Autodesk Fusion 360 part; units mm, degrees
note: some values were not read from the file. Chosen so that the rebuilt part matches the saved one: which bodies a step acts on.
(part 2 of 2)
sketch "Sketch6" plane through (0, 3, 0) normal (0, 1, 0) x (-1, 0, 0)
  line L0 (-6.1781, 100.7305) -> (-1.9988, 100.5953)
  line L1 (-1.9988, 100.5953) -> (-0.8032, 103.5868)
  line L2 (-0.8032, 103.5868) -> (0.6012, 103.5414)
  line L3 (0.6012, 103.5414) -> (-3.5606, 93.6708)
  line L4 (-3.5606, 93.6708) -> (-4.9855, 93.717)
  line L5 (-4.9855, 93.717) -> (-8.7527, 103.8441)
  line L6 (-8.7527, 103.8441) -> (-7.246, 103.7953)
  line L7 (-7.246, 103.7953) -> (-6.1781, 100.7305)
  spline S0 degree 2 poles (18.1316, 102.5774) (18.5781, 102.8912) (19.2412, 103.038) knots 0 0 0 1 1 1
  spline S1 degree 2 poles (19.2412, 103.038) (19.9043, 103.1848) (20.8588, 103.1554) knots 0 0 0 1 1 1
  line L8 (20.8588, 103.1554) -> (24.6701, 103.0379)
  line L9 (24.6701, 103.0379) -> (24.3621, 93.0427)
  line L10 (24.3621, 93.0427) -> (20.6122, 93.1582)
  spline S2 degree 2 poles (20.6122, 93.1582) (19.4667, 93.1935) (18.784, 93.5182) knots 0 0 0 1 1 1
  spline S3 degree 2 poles (18.784, 93.5182) (18.1014, 93.843) (17.7288, 94.4857) knots 0 0 0 1 1 1
  spline S4 degree 2 poles (17.7288, 94.4857) (17.3562, 95.1285) (17.3774, 95.8171) knots 0 0 0 1 1 1
  spline S5 degree 2 poles (17.3774, 95.8171) (17.3971, 96.458) (17.7623, 97.0132) knots 0 0 0 1 1 1
  spline S6 degree 2 poles (17.7623, 97.0132) (18.1274, 97.5683) (18.8404, 97.8944) knots 0 0 0 1 1 1
  spline S7 degree 2 poles (18.8404, 97.8944) (17.9418, 98.1883) (17.4741, 98.8442) knots 0 0 0 1 1 1
  spline S8 degree 2 poles (17.4741, 98.8442) (17.0063, 99.5001) (17.0332, 100.3728) knots 0 0 0 1 1 1
  spline S9 degree 2 poles (17.0332, 100.3728) (17.0548, 101.0751) (17.37, 101.6693) knots 0 0 0 1 1 1
  spline S10 degree 2 poles (17.37, 101.6693) (17.6852, 102.2636) (18.1316, 102.5774) knots 0 0 0 1 1 1
  line L11 (9.2769, 96.8199) -> (3.1378, 96.8199)
  line L12 (3.1378, 96.8199) -> (3.1378, 98)
  line L13 (3.1378, 98) -> (10.6003, 98)
  line L14 (10.6003, 98) -> (10.6003, 88)
  line L15 (10.6003, 88) -> (3.3697, 88)
  line L16 (3.3697, 88) -> (3.3697, 89.1801)
  line L17 (3.3697, 89.1801) -> (9.2769, 89.1801)
  line L18 (9.2769, 89.1801) -> (9.2769, 92.2428)
  line L19 (9.2769, 92.2428) -> (3.7449, 92.2428)
  line L20 (3.7449, 92.2428) -> (3.7449, 93.4161)
  line L21 (3.7449, 93.4161) -> (9.2769, 93.4161)
  line L22 (9.2769, 93.4161) -> (9.2769, 96.8199)
  circle A0 centre (0, 10) radius 1.5
  circle A1 centre (18.755, -13.3979) radius 1.5
  circle A2 centre (-50, 20) radius 1.5
  circle A3 centre (50, 10) radius 1.5
  circle A4 centre (19.4752, -45.0876) radius 1.5
  circle A5 centre (30, -66.3341) radius 1.5
  circle A6 centre (50, 80) radius 1.5
  circle A7 centre (-20, 20) radius 1.5
  circle A8 centre (-20.1369, -46.1679) radius 1.5
  circle A9 centre (-29.8599, -66.6942) radius 1.5
  circle A10 centre (0, 80) radius 1.5
  circle A11 centre (-20.8571, -13.7581) radius 1.5
  arc A12 (60, 0) -> (30, -30) centre (60, -30) ccw
  line L23 (60, 0) -> (60, 60)
  line L24 (60, 60) -> (70, 70)
  line L25 (70, 70) -> (70, 110)
  line L26 (70, 110) -> (-70, 110)
  line L27 (-70, 110) -> (-70, 70)
  line L28 (-70, 70) -> (-60, 60)
  line L29 (-60, 60) -> (-60, 0)
  arc A13 (-30, -30) -> (-60, 0) centre (-60, -30) ccw
  line L30 (-30, -30) -> (-30, -60)
  line L31 (-30, -60) -> (-60, -40)
  line L32 (-60, -40) -> (-60, -80)
  line L33 (-60, -80) -> (-30, -80)
  line L34 (-30, -80) -> (0, -100)
  line L35 (0, -100) -> (30, -80)
  line L36 (30, -80) -> (60, -80)
  line L37 (60, -80) -> (60, -40)
  line L38 (60, -40) -> (30, -60)
  line L39 (30, -60) -> (30, -30)
  line L40 (-15.3458, 97.2305) -> (-13.811, 97.2305)
  line L41 (-13.811, 97.2305) -> (-13.811, 101.6712)
  line L42 (-13.811, 101.6712) -> (-12.4876, 101.6712)
  line L43 (-12.4876, 101.6712) -> (-12.4876, 91.6712)
  line L44 (-12.4876, 91.6712) -> (-16.9215, 91.6712)
  spline S11 degree 2 poles (-16.9215, 91.6712) (-18.2585, 91.6712) (-18.9542, 91.9406) knots 0 0 0 1 1 1
  spline S12 degree 2 poles (-18.9542, 91.9406) (-19.65, 92.2101) (-20.0661, 92.8922) knots 0 0 0 1 1 1
  spline S13 degree 2 poles (-20.0661, 92.8922) (-20.4822, 93.5743) (-20.4822, 94.3997) knots 0 0 0 1 1 1
  spline S14 degree 2 poles (-20.4822, 94.3997) (-20.4822, 95.4638) (-19.7932, 96.1937) knots 0 0 0 1 1 1
  spline S15 degree 2 poles (-19.7932, 96.1937) (-19.1043, 96.9236) (-17.665, 97.1214) knots 0 0 0 1 1 1
  spline S16 degree 2 poles (-17.665, 97.1214) (-18.1902, 97.3738) (-18.4631, 97.6193) knots 0 0 0 1 1 1
  spline S17 degree 2 poles (-18.4631, 97.6193) (-19.0429, 98.1514) (-19.5613, 98.9495) knots 0 0 0 1 1 1
  line L45 (-19.5613, 98.9495) -> (-21.3007, 101.6712)
  line L46 (-21.3007, 101.6712) -> (-19.6364, 101.6712)
  line L47 (-19.6364, 101.6712) -> (-18.313, 99.5907)
  spline S18 degree 2 poles (-18.313, 99.5907) (-17.7332, 98.6903) (-17.358, 98.2128) knots 0 0 0 1 1 1
  spline S19 degree 2 poles (-17.358, 98.2128) (-16.9829, 97.7353) (-16.6861, 97.5443) knots 0 0 0 1 1 1
  spline S20 degree 2 poles (-16.6861, 97.5443) (-16.3894, 97.3533) (-16.0825, 97.2783) knots 0 0 0 1 1 1
  spline S21 degree 2 poles (-16.0825, 97.2783) (-15.8574, 97.2305) (-15.3458, 97.2305) knots 0 0 0 1 1 1
  line L48 (-24.0007, 95.7872) -> (-25.249, 95.6779)
  spline S22 degree 2 poles (-25.249, 95.6779) (-25.3378, 96.4282) (-25.6618, 96.9091) knots 0 0 0 1 1 1
  spline S23 degree 2 poles (-25.6618, 96.9091) (-25.9859, 97.39) (-26.6681, 97.6866) knots 0 0 0 1 1 1
  spline S24 degree 2 poles (-26.6681, 97.6866) (-27.3502, 97.9833) (-28.2029, 97.9832) knots 0 0 0 1 1 1
  spline S25 degree 2 poles (-28.2029, 97.9832) (-28.96, 97.9831) (-29.5398, 97.7579) knots 0 0 0 1 1 1
  spline S26 degree 2 poles (-29.5398, 97.7579) (-30.1196, 97.5328) (-30.4027, 97.1405) knots 0 0 0 1 1 1
  spline S27 degree 2 poles (-30.4027, 97.1405) (-30.6857, 96.7483) (-30.6856, 96.2844) knots 0 0 0 1 1 1
  spline S28 degree 2 poles (-30.6856, 96.2844) (-30.6856, 95.8137) (-30.4127, 95.4625) knots 0 0 0 1 1 1
  spline S29 degree 2 poles (-30.4127, 95.4625) (-30.1398, 95.1112) (-29.5122, 94.8725) knots 0 0 0 1 1 1
  spline S30 degree 2 poles (-29.5122, 94.8725) (-29.1098, 94.7157) (-27.7318, 94.385) knots 0 0 0 1 1 1
  spline S31 degree 2 poles (-27.7318, 94.385) (-26.3539, 94.0543) (-25.8013, 93.7611) knots 0 0 0 1 1 1
  spline S32 degree 2 poles (-25.8013, 93.7611) (-25.0851, 93.386) (-24.7337, 92.8301) knots 0 0 0 1 1 1
  spline S33 degree 2 poles (-24.7337, 92.8301) (-24.3823, 92.2742) (-24.3823, 91.5852) knots 0 0 0 1 1 1
  spline S34 degree 2 poles (-24.3823, 91.5852) (-24.3822, 90.8281) (-24.8119, 90.1698) knots 0 0 0 1 1 1
  spline S35 degree 2 poles (-24.8119, 90.1698) (-25.2415, 89.5115) (-26.0669, 89.1703) knots 0 0 0 1 1 1
  spline S36 degree 2 poles (-26.0669, 89.1703) (-26.8922, 88.8292) (-27.9018, 88.829) knots 0 0 0 1 1 1
  spline S37 degree 2 poles (-27.9018, 88.829) (-29.0136, 88.8289) (-29.8629, 89.187) knots 0 0 0 1 1 1
  spline S38 degree 2 poles (-29.8629, 89.187) (-30.7122, 89.545) (-31.1693, 90.2407) knots 0 0 0 1 1 1
  spline S39 degree 2 poles (-31.1693, 90.2407) (-31.6264, 90.9364) (-31.6606, 91.8164) knots 0 0 0 1 1 1
  line L49 (-31.6606, 91.8164) -> (-30.3919, 91.912)
  spline S40 degree 2 poles (-30.3919, 91.912) (-30.2894, 90.9639) (-29.6993, 90.4796) knots 0 0 0 1 1 1
  spline S41 degree 2 poles (-29.6993, 90.4796) (-29.1092, 89.9954) (-27.9565, 89.9955) knots 0 0 0 1 1 1
  spline S42 degree 2 poles (-27.9565, 89.9955) (-26.7559, 89.9956) (-26.2068, 90.4356) knots 0 0 0 1 1 1
  spline S43 degree 2 poles (-26.2068, 90.4356) (-25.6578, 90.8757) (-25.6578, 91.4964) knots 0 0 0 1 1 1
  spline S44 degree 2 poles (-25.6578, 91.4964) (-25.6579, 92.0353) (-26.0468, 92.3831) knots 0 0 0 1 1 1
  spline S45 degree 2 poles (-26.0468, 92.3831) (-26.4288, 92.731) (-28.0421, 93.0957) knots 0 0 0 1 1 1
  spline S46 degree 2 poles (-28.0421, 93.0957) (-29.6553, 93.4605) (-30.2556, 93.7333) knots 0 0 0 1 1 1
  spline S47 degree 2 poles (-30.2556, 93.7333) (-31.1288, 94.1357) (-31.545, 94.7529) knots 0 0 0 1 1 1
  spline S48 degree 2 poles (-31.545, 94.7529) (-31.9611, 95.3702) (-31.9612, 96.1751) knots 0 0 0 1 1 1
  spline S49 degree 2 poles (-31.9612, 96.1751) (-31.9613, 96.9732) (-31.5043, 97.6793) knots 0 0 0 1 1 1
  spline S50 degree 2 poles (-31.5043, 97.6793) (-31.0474, 98.3853) (-30.1914, 98.7776) knots 0 0 0 1 1 1
  spline S51 degree 2 poles (-30.1914, 98.7776) (-29.3353, 99.17) (-28.2644, 99.1701) knots 0 0 0 1 1 1
  spline S52 degree 2 poles (-28.2644, 99.1701) (-26.907, 99.1702) (-25.9895, 98.7747) knots 0 0 0 1 1 1
  spline S53 degree 2 poles (-25.9895, 98.7747) (-25.072, 98.3791) (-24.55, 97.5845) knots 0 0 0 1 1 1
  spline S54 degree 2 poles (-24.55, 97.5845) (-24.0281, 96.7899) (-24.0007, 95.7872) knots 0 0 0 1 1 1
extrude "Extrude6" cut sketch "Sketch6" against normal blind 3 contours L48 S22 S23 S24 S25 S26 S27 S28 S29 S30 S31 S32 S33 S34 S35 S36 S37 S38 S39 L49 S40 S41 S42 S43 S44 S45 S46 S47 S48 S49 S50 S51 S52 S53 S54 bodies 10
sketch "Sketch7" plane through (0, 3, 0) normal (0, 1, 0) x (-1, 0, 0)
  spline S0 degree 2 poles (-28.2644, 99.1701) (-26.907, 99.1702) (-25.9895, 98.7747) knots 0 0 0 1 1 1
  spline S1 degree 2 poles (-25.9895, 98.7747) (-25.072, 98.3791) (-24.55, 97.5845) knots 0 0 0 1 1 1
  spline S2 degree 2 poles (-24.55, 97.5845) (-24.0281, 96.7899) (-24.0007, 95.7872) knots 0 0 0 1 1 1
  line L0 (-24.0007, 95.7872) -> (-25.249, 95.6779)
  spline S3 degree 2 poles (-25.249, 95.6779) (-25.3378, 96.4282) (-25.6618, 96.9091) knots 0 0 0 1 1 1
  spline S4 degree 2 poles (-25.6618, 96.9091) (-25.9859, 97.39) (-26.6681, 97.6866) knots 0 0 0 1 1 1
  spline S5 degree 2 poles (-26.6681, 97.6866) (-27.3502, 97.9833) (-28.2029, 97.9832) knots 0 0 0 1 1 1
  spline S6 degree 2 poles (-28.2029, 97.9832) (-28.96, 97.9831) (-29.5398, 97.7579) knots 0 0 0 1 1 1
  spline S7 degree 2 poles (-29.5398, 97.7579) (-30.1196, 97.5328) (-30.4027, 97.1405) knots 0 0 0 1 1 1
  spline S8 degree 2 poles (-30.4027, 97.1405) (-30.6857, 96.7483) (-30.6856, 96.2844) knots 0 0 0 1 1 1
  spline S9 degree 2 poles (-30.6856, 96.2844) (-30.6856, 95.8137) (-30.4127, 95.4625) knots 0 0 0 1 1 1
  spline S10 degree 2 poles (-30.4127, 95.4625) (-30.1398, 95.1112) (-29.5122, 94.8725) knots 0 0 0 1 1 1
  spline S11 degree 2 poles (-29.5122, 94.8725) (-29.1098, 94.7157) (-27.7318, 94.385) knots 0 0 0 1 1 1
  spline S12 degree 2 poles (-27.7318, 94.385) (-26.3539, 94.0543) (-25.8013, 93.7611) knots 0 0 0 1 1 1
  spline S13 degree 2 poles (-25.8013, 93.7611) (-25.0851, 93.386) (-24.7337, 92.8301) knots 0 0 0 1 1 1
  spline S14 degree 2 poles (-24.7337, 92.8301) (-24.3823, 92.2742) (-24.3823, 91.5852) knots 0 0 0 1 1 1
  spline S15 degree 2 poles (-24.3823, 91.5852) (-24.3822, 90.8281) (-24.8119, 90.1698) knots 0 0 0 1 1 1
  spline S16 degree 2 poles (-24.8119, 90.1698) (-25.2415, 89.5115) (-26.0669, 89.1703) knots 0 0 0 1 1 1
  spline S17 degree 2 poles (-26.0669, 89.1703) (-26.8922, 88.8292) (-27.9018, 88.829) knots 0 0 0 1 1 1
  spline S18 degree 2 poles (-27.9018, 88.829) (-29.0136, 88.8289) (-29.8629, 89.187) knots 0 0 0 1 1 1
  spline S19 degree 2 poles (-29.8629, 89.187) (-30.7122, 89.545) (-31.1693, 90.2407) knots 0 0 0 1 1 1
  spline S20 degree 2 poles (-31.1693, 90.2407) (-31.6264, 90.9364) (-31.6606, 91.8164) knots 0 0 0 1 1 1
  line L1 (-31.6606, 91.8164) -> (-30.3919, 91.912)
  spline S21 degree 2 poles (-30.3919, 91.912) (-30.2894, 90.9639) (-29.6993, 90.4796) knots 0 0 0 1 1 1
  spline S22 degree 2 poles (-29.6993, 90.4796) (-29.1092, 89.9954) (-27.9565, 89.9955) knots 0 0 0 1 1 1
  spline S23 degree 2 poles (-27.9565, 89.9955) (-26.7559, 89.9956) (-26.2068, 90.4356) knots 0 0 0 1 1 1
  spline S24 degree 2 poles (-26.2068, 90.4356) (-25.6578, 90.8757) (-25.6578, 91.4964) knots 0 0 0 1 1 1
  spline S25 degree 2 poles (-25.6578, 91.4964) (-25.6579, 92.0353) (-26.0468, 92.3831) knots 0 0 0 1 1 1
  spline S26 degree 2 poles (-26.0468, 92.3831) (-26.4288, 92.731) (-28.0421, 93.0957) knots 0 0 0 1 1 1
  spline S27 degree 2 poles (-28.0421, 93.0957) (-29.6553, 93.4605) (-30.2556, 93.7333) knots 0 0 0 1 1 1
  spline S28 degree 2 poles (-30.2556, 93.7333) (-31.1288, 94.1357) (-31.545, 94.7529) knots 0 0 0 1 1 1
  spline S29 degree 2 poles (-31.545, 94.7529) (-31.9611, 95.3702) (-31.9612, 96.1751) knots 0 0 0 1 1 1
  spline S30 degree 2 poles (-31.9612, 96.1751) (-31.9613, 96.9732) (-31.5043, 97.6793) knots 0 0 0 1 1 1
  spline S31 degree 2 poles (-31.5043, 97.6793) (-31.0474, 98.3853) (-30.1914, 98.7776) knots 0 0 0 1 1 1
  spline S32 degree 2 poles (-30.1914, 98.7776) (-29.3353, 99.17) (-28.2644, 99.1701) knots 0 0 0 1 1 1
  line L2 (-6.1781, 100.7305) -> (-1.9988, 100.5953)
  line L3 (-1.9988, 100.5953) -> (-0.8032, 103.5868)
  line L4 (-0.8032, 103.5868) -> (0.6012, 103.5414)
  line L5 (0.6012, 103.5414) -> (-3.5606, 93.6708)
  line L6 (-3.5606, 93.6708) -> (-4.9855, 93.717)
  line L7 (-4.9855, 93.717) -> (-8.7527, 103.8441)
  line L8 (-8.7527, 103.8441) -> (-7.246, 103.7953)
  line L9 (-7.246, 103.7953) -> (-6.1781, 100.7305)
  spline S33 degree 2 poles (18.1316, 102.5774) (18.5781, 102.8912) (19.2412, 103.038) knots 0 0 0 1 1 1
  spline S34 degree 2 poles (19.2412, 103.038) (19.9043, 103.1848) (20.8588, 103.1554) knots 0 0 0 1 1 1
  line L10 (20.8588, 103.1554) -> (24.6701, 103.0379)
  line L11 (24.6701, 103.0379) -> (24.3621, 93.0427)
  line L12 (24.3621, 93.0427) -> (20.6122, 93.1582)
  spline S35 degree 2 poles (20.6122, 93.1582) (19.4667, 93.1935) (18.784, 93.5182) knots 0 0 0 1 1 1
  spline S36 degree 2 poles (18.784, 93.5182) (18.1014, 93.843) (17.7288, 94.4857) knots 0 0 0 1 1 1
  spline S37 degree 2 poles (17.7288, 94.4857) (17.3562, 95.1285) (17.3774, 95.8171) knots 0 0 0 1 1 1
  spline S38 degree 2 poles (17.3774, 95.8171) (17.3971, 96.458) (17.7623, 97.0132) knots 0 0 0 1 1 1
  spline S39 degree 2 poles (17.7623, 97.0132) (18.1274, 97.5683) (18.8404, 97.8944) knots 0 0 0 1 1 1
  spline S40 degree 2 poles (18.8404, 97.8944) (17.9418, 98.1883) (17.4741, 98.8442) knots 0 0 0 1 1 1
  spline S41 degree 2 poles (17.4741, 98.8442) (17.0063, 99.5001) (17.0332, 100.3728) knots 0 0 0 1 1 1
  spline S42 degree 2 poles (17.0332, 100.3728) (17.0548, 101.0751) (17.37, 101.6693) knots 0 0 0 1 1 1
  spline S43 degree 2 poles (17.37, 101.6693) (17.6852, 102.2636) (18.1316, 102.5774) knots 0 0 0 1 1 1
  line L13 (9.2769, 96.8199) -> (3.1378, 96.8199)
  line L14 (3.1378, 96.8199) -> (3.1378, 98)
  line L15 (3.1378, 98) -> (10.6003, 98)
  line L16 (10.6003, 98) -> (10.6003, 88)
  line L17 (10.6003, 88) -> (3.3697, 88)
  line L18 (3.3697, 88) -> (3.3697, 89.1801)
  line L19 (3.3697, 89.1801) -> (9.2769, 89.1801)
  line L20 (9.2769, 89.1801) -> (9.2769, 92.2428)
  line L21 (9.2769, 92.2428) -> (3.7449, 92.2428)
  line L22 (3.7449, 92.2428) -> (3.7449, 93.4161)
  line L23 (3.7449, 93.4161) -> (9.2769, 93.4161)
  line L24 (9.2769, 93.4161) -> (9.2769, 96.8199)
  circle A0 centre (0, 10) radius 1.5
  circle A1 centre (18.755, -13.3979) radius 1.5
  circle A2 centre (-50, 20) radius 1.5
  circle A3 centre (50, 10) radius 1.5
  circle A4 centre (19.4752, -45.0876) radius 1.5
  circle A5 centre (30, -66.3341) radius 1.5
  circle A6 centre (50, 80) radius 1.5
  circle A7 centre (-20, 20) radius 1.5
  circle A8 centre (-20.1369, -46.1679) radius 1.5
  circle A9 centre (-29.8599, -66.6942) radius 1.5
  circle A10 centre (0, 80) radius 1.5
  circle A11 centre (-20.8571, -13.7581) radius 1.5
  arc A12 (60, 0) -> (30, -30) centre (60, -30) ccw
  line L25 (60, 0) -> (60, 60)
  line L26 (60, 60) -> (70, 70)
  line L27 (70, 70) -> (70, 110)
  line L28 (70, 110) -> (-70, 110)
  line L29 (-70, 110) -> (-70, 70)
  line L30 (-70, 70) -> (-60, 60)
  line L31 (-60, 60) -> (-60, 0)
  arc A13 (-30, -30) -> (-60, 0) centre (-60, -30) ccw
  line L32 (-30, -30) -> (-30, -60)
  line L33 (-30, -60) -> (-60, -40)
  line L34 (-60, -40) -> (-60, -80)
  line L35 (-60, -80) -> (-30, -80)
  line L36 (-30, -80) -> (0, -100)
  line L37 (0, -100) -> (30, -80)
  line L38 (30, -80) -> (60, -80)
  line L39 (60, -80) -> (60, -40)
  line L40 (60, -40) -> (30, -60)
  line L41 (30, -60) -> (30, -30)
  line L42 (-15.3458, 97.2305) -> (-13.811, 97.2305)
  line L43 (-13.811, 97.2305) -> (-13.811, 101.6712)
  line L44 (-13.811, 101.6712) -> (-12.4876, 101.6712)
  line L45 (-12.4876, 101.6712) -> (-12.4876, 91.6712)
  line L46 (-12.4876, 91.6712) -> (-16.9215, 91.6712)
  spline S44 degree 2 poles (-16.9215, 91.6712) (-18.2585, 91.6712) (-18.9542, 91.9406) knots 0 0 0 1 1 1
  spline S45 degree 2 poles (-18.9542, 91.9406) (-19.65, 92.2101) (-20.0661, 92.8922) knots 0 0 0 1 1 1
  spline S46 degree 2 poles (-20.0661, 92.8922) (-20.4822, 93.5743) (-20.4822, 94.3997) knots 0 0 0 1 1 1
  spline S47 degree 2 poles (-20.4822, 94.3997) (-20.4822, 95.4638) (-19.7932, 96.1937) knots 0 0 0 1 1 1
  spline S48 degree 2 poles (-19.7932, 96.1937) (-19.1043, 96.9236) (-17.665, 97.1214) knots 0 0 0 1 1 1
  spline S49 degree 2 poles (-17.665, 97.1214) (-18.1902, 97.3738) (-18.4631, 97.6193) knots 0 0 0 1 1 1
  spline S50 degree 2 poles (-18.4631, 97.6193) (-19.0429, 98.1514) (-19.5613, 98.9495) knots 0 0 0 1 1 1
  line L47 (-19.5613, 98.9495) -> (-21.3007, 101.6712)
  line L48 (-21.3007, 101.6712) -> (-19.6364, 101.6712)
  line L49 (-19.6364, 101.6712) -> (-18.313, 99.5907)
  spline S51 degree 2 poles (-18.313, 99.5907) (-17.7332, 98.6903) (-17.358, 98.2128) knots 0 0 0 1 1 1
  spline S52 degree 2 poles (-17.358, 98.2128) (-16.9829, 97.7353) (-16.6861, 97.5443) knots 0 0 0 1 1 1
  spline S53 degree 2 poles (-16.6861, 97.5443) (-16.3894, 97.3533) (-16.0825, 97.2783) knots 0 0 0 1 1 1
  spline S54 degree 2 poles (-16.0825, 97.2783) (-15.8574, 97.2305) (-15.3458, 97.2305) knots 0 0 0 1 1 1
  line L50 (25, 150) -> (25, 140)
  line L51 (25, 140) -> (21.2483, 140)
  spline S55 degree 2 poles (21.2483, 140) (20.1023, 140) (19.41, 140.3035) knots 0 0 0 1 1 1
  spline S56 degree 2 poles (19.41, 140.3035) (18.7176, 140.6071) (18.3254, 141.2381) knots 0 0 0 1 1 1
  spline S57 degree 2 poles (18.3254, 141.2381) (17.9332, 141.869) (17.9332, 142.558) knots 0 0 0 1 1 1
  spline S58 degree 2 poles (17.9332, 142.558) (17.9332, 143.1992) (18.281, 143.7653) knots 0 0 0 1 1 1
  spline S59 degree 2 poles (18.281, 143.7653) (18.6289, 144.3315) (19.3315, 144.6794) knots 0 0 0 1 1 1
  spline S60 degree 2 poles (19.3315, 144.6794) (18.4243, 144.9454) (17.9366, 145.5866) knots 0 0 0 1 1 1
  spline S61 degree 2 poles (17.9366, 145.5866) (17.4488, 146.2278) (17.4488, 147.101) knots 0 0 0 1 1 1
  spline S62 degree 2 poles (17.4488, 147.101) (17.4488, 147.8035) (17.7456, 148.4072) knots 0 0 0 1 1 1
  spline S63 degree 2 poles (17.7456, 148.4072) (18.0423, 149.0109) (18.4789, 149.3383) knots 0 0 0 1 1 1
  spline S64 degree 2 poles (18.4789, 149.3383) (18.9154, 149.6658) (19.5737, 149.8329) knots 0 0 0 1 1 1
  spline S65 degree 2 poles (19.5737, 149.8329) (20.2319, 150) (21.1869, 150) knots 0 0 0 1 1 1
  line L52 (21.1869, 150) -> (25, 150)
  line L53 (23.6767, 144.2019) -> (21.5143, 144.2019)
  spline S66 degree 2 poles (21.5143, 144.2019) (20.6344, 144.2019) (20.2524, 144.0859) knots 0 0 0 1 1 1
  spline S67 degree 2 poles (20.2524, 144.0859) (19.7476, 143.9359) (19.4918, 143.588) knots 0 0 0 1 1 1
  spline S68 degree 2 poles (19.4918, 143.588) (19.236, 143.2401) (19.236, 142.7149) knots 0 0 0 1 1 1
  spline S69 degree 2 poles (19.236, 142.7149) (19.236, 142.2169) (19.4748, 141.8383) knots 0 0 0 1 1 1
  spline S70 degree 2 poles (19.4748, 141.8383) (19.7135, 141.4598) (20.1569, 141.3199) knots 0 0 0 1 1 1
  spline S71 degree 2 poles (20.1569, 141.3199) (20.6003, 141.1801) (21.678, 141.1801) knots 0 0 0 1 1 1
  line L54 (21.678, 141.1801) -> (23.6767, 141.1801)
  line L55 (23.6767, 141.1801) -> (23.6767, 144.2019)
  line L56 (23.6767, 148.8199) -> (21.1869, 148.8199)
  spline S72 degree 2 poles (21.1869, 148.8199) (20.5457, 148.8199) (20.2865, 148.7722) knots 0 0 0 1 1 1
  spline S73 degree 2 poles (20.2865, 148.7722) (19.8295, 148.6903) (19.5225, 148.4993) knots 0 0 0 1 1 1
  spline S74 degree 2 poles (19.5225, 148.4993) (19.2156, 148.3083) (19.0177, 147.9434) knots 0 0 0 1 1 1
  spline S75 degree 2 poles (19.0177, 147.9434) (18.8199, 147.5784) (18.8199, 147.101) knots 0 0 0 1 1 1
  spline S76 degree 2 poles (18.8199, 147.101) (18.8199, 146.5416) (19.1064, 146.1289) knots 0 0 0 1 1 1
  spline S77 degree 2 poles (19.1064, 146.1289) (19.3929, 145.7162) (19.9011, 145.5491) knots 0 0 0 1 1 1
  spline S78 degree 2 poles (19.9011, 145.5491) (20.4093, 145.382) (21.3643, 145.382) knots 0 0 0 1 1 1
  line L57 (21.3643, 145.382) -> (23.6767, 145.382)
  line L58 (23.6767, 145.382) -> (23.6767, 148.8199)
  line L59 (15.6003, 150) -> (15.6003, 140)
  line L60 (15.6003, 140) -> (8.3697, 140)
  line L61 (8.3697, 140) -> (8.3697, 141.1801)
  line L62 (8.3697, 141.1801) -> (14.2769, 141.1801)
  line L63 (14.2769, 141.1801) -> (14.2769, 144.2428)
  line L64 (14.2769, 144.2428) -> (8.7449, 144.2428)
  line L65 (8.7449, 144.2428) -> (8.7449, 145.4161)
  line L66 (8.7449, 145.4161) -> (14.2769, 145.4161)
  line L67 (14.2769, 145.4161) -> (14.2769, 148.8199)
  line L68 (14.2769, 148.8199) -> (8.1378, 148.8199)
  line L69 (8.1378, 148.8199) -> (8.1378, 150)
  line L70 (8.1378, 150) -> (15.6003, 150)
  line L71 (7.4079, 150) -> (3.5675, 140)
  line L72 (3.5675, 140) -> (2.1419, 140)
  line L73 (2.1419, 140) -> (-1.9509, 150)
  line L74 (-1.9509, 150) -> (-0.4434, 150)
  line L75 (-0.4434, 150) -> (0.7231, 146.9714)
  line L76 (0.7231, 146.9714) -> (4.9045, 146.9714)
  line L77 (4.9045, 146.9714) -> (6.0027, 150)
  line L78 (6.0027, 150) -> (7.4079, 150)
  line L79 (4.5225, 145.8936) -> (1.1323, 145.8936)
  line L80 (1.1323, 145.8936) -> (2.176, 143.1241)
  spline S79 degree 2 poles (2.176, 143.1241) (2.6535, 141.8622) (2.8854, 141.0505) knots 0 0 0 1 1 1
  spline S80 degree 2 poles (2.8854, 141.0505) (3.0764, 142.0123) (3.4243, 142.9604) knots 0 0 0 1 1 1
  line L81 (3.4243, 142.9604) -> (4.5225, 145.8936)
  line L82 (-3.0287, 150) -> (-3.0287, 140)
  line L83 (-3.0287, 140) -> (-7.4625, 140)
  spline S81 degree 2 poles (-7.4625, 140) (-8.7995, 140) (-9.4952, 140.2694) knots 0 0 0 1 1 1
  spline S82 degree 2 poles (-9.4952, 140.2694) (-10.191, 140.5389) (-10.6071, 141.221) knots 0 0 0 1 1 1
  spline S83 degree 2 poles (-10.6071, 141.221) (-11.0232, 141.9031) (-11.0232, 142.7285) knots 0 0 0 1 1 1
  spline S84 degree 2 poles (-11.0232, 142.7285) (-11.0232, 143.7926) (-10.3342, 144.5225) knots 0 0 0 1 1 1
  spline S85 degree 2 poles (-10.3342, 144.5225) (-9.6453, 145.2524) (-8.206, 145.4502) knots 0 0 0 1 1 1
  spline S86 degree 2 poles (-8.206, 145.4502) (-8.7312, 145.7026) (-9.0041, 145.9482) knots 0 0 0 1 1 1
  spline S87 degree 2 poles (-9.0041, 145.9482) (-9.5839, 146.4802) (-10.1023, 147.2783) knots 0 0 0 1 1 1
  line L84 (-10.1023, 147.2783) -> (-11.8417, 150)
  line L85 (-11.8417, 150) -> (-10.1774, 150)
  line L86 (-10.1774, 150) -> (-8.854, 147.9195)
  spline S88 degree 2 poles (-8.854, 147.9195) (-8.2742, 147.0191) (-7.899, 146.5416) knots 0 0 0 1 1 1
  spline S89 degree 2 poles (-7.899, 146.5416) (-7.5239, 146.0641) (-7.2271, 145.8731) knots 0 0 0 1 1 1
  spline S90 degree 2 poles (-7.2271, 145.8731) (-6.9304, 145.6821) (-6.6235, 145.6071) knots 0 0 0 1 1 1
  spline S91 degree 2 poles (-6.6235, 145.6071) (-6.3984, 145.5593) (-5.8868, 145.5593) knots 0 0 0 1 1 1
  line L87 (-5.8868, 145.5593) -> (-4.352, 145.5593)
  line L88 (-4.352, 145.5593) -> (-4.352, 150)
  line L89 (-4.352, 150) -> (-3.0287, 150)
  line L90 (-4.352, 144.4134) -> (-7.1965, 144.4134)
  spline S92 degree 2 poles (-7.1965, 144.4134) (-8.1037, 144.4134) (-8.6153, 144.2258) knots 0 0 0 1 1 1
  spline S93 degree 2 poles (-8.6153, 144.2258) (-9.1269, 144.0382) (-9.3929, 143.6255) knots 0 0 0 1 1 1
  spline S94 degree 2 poles (-9.3929, 143.6255) (-9.6589, 143.2128) (-9.6589, 142.7285) knots 0 0 0 1 1 1
  spline S95 degree 2 poles (-9.6589, 142.7285) (-9.6589, 142.0191) (-9.1439, 141.5621) knots 0 0 0 1 1 1
  spline S96 degree 2 poles (-9.1439, 141.5621) (-8.6289, 141.105) (-7.5171, 141.105) knots 0 0 0 1 1 1
  line L91 (-7.5171, 141.105) -> (-4.352, 141.105)
  line L92 (-4.352, 141.105) -> (-4.352, 144.4134)
  line L93 (-12.6467, 146.7872) -> (-13.895, 146.678)
  spline S97 degree 2 poles (-13.895, 146.678) (-13.9836, 147.4284) (-14.3076, 147.9093) knots 0 0 0 1 1 1
  spline S98 degree 2 poles (-14.3076, 147.9093) (-14.6317, 148.3902) (-15.3138, 148.6869) knots 0 0 0 1 1 1
  spline S99 degree 2 poles (-15.3138, 148.6869) (-15.9959, 148.9836) (-16.8486, 148.9836) knots 0 0 0 1 1 1
  spline S100 degree 2 poles (-16.8486, 148.9836) (-17.6057, 148.9836) (-18.1855, 148.7585) knots 0 0 0 1 1 1
  spline S101 degree 2 poles (-18.1855, 148.7585) (-18.7653, 148.5334) (-19.0484, 148.1412) knots 0 0 0 1 1 1
  spline S102 degree 2 poles (-19.0484, 148.1412) (-19.3315, 147.749) (-19.3315, 147.2851) knots 0 0 0 1 1 1
  spline S103 degree 2 poles (-19.3315, 147.2851) (-19.3315, 146.8145) (-19.0587, 146.4632) knots 0 0 0 1 1 1
  spline S104 degree 2 poles (-19.0587, 146.4632) (-18.7858, 146.1119) (-18.1583, 145.8731) knots 0 0 0 1 1 1
  spline S105 degree 2 poles (-18.1583, 145.8731) (-17.7558, 145.7162) (-16.3779, 145.3854) knots 0 0 0 1 1 1
  spline S106 degree 2 poles (-16.3779, 145.3854) (-15, 145.0546) (-14.4475, 144.7613) knots 0 0 0 1 1 1
  spline S107 degree 2 poles (-14.4475, 144.7613) (-13.7312, 144.3861) (-13.3799, 143.8302) knots 0 0 0 1 1 1
  spline S108 degree 2 poles (-13.3799, 143.8302) (-13.0287, 143.2742) (-13.0287, 142.5853) knots 0 0 0 1 1 1
  spline S109 degree 2 poles (-13.0287, 142.5853) (-13.0287, 141.8281) (-13.4584, 141.1699) knots 0 0 0 1 1 1
  spline S110 degree 2 poles (-13.4584, 141.1699) (-13.8881, 140.5116) (-14.7135, 140.1705) knots 0 0 0 1 1 1
  spline S111 degree 2 poles (-14.7135, 140.1705) (-15.5389, 139.8295) (-16.5484, 139.8295) knots 0 0 0 1 1 1
  spline S112 degree 2 poles (-16.5484, 139.8295) (-17.6603, 139.8295) (-18.5096, 140.1876) knots 0 0 0 1 1 1
  spline S113 degree 2 poles (-18.5096, 140.1876) (-19.3588, 140.5457) (-19.8158, 141.2415) knots 0 0 0 1 1 1
  spline S114 degree 2 poles (-19.8158, 141.2415) (-20.2729, 141.9372) (-20.307, 142.8172) knots 0 0 0 1 1 1
  line L94 (-20.307, 142.8172) -> (-19.0382, 142.9127)
  spline S115 degree 2 poles (-19.0382, 142.9127) (-18.9359, 141.9645) (-18.3458, 141.4802) knots 0 0 0 1 1 1
  spline S116 degree 2 poles (-18.3458, 141.4802) (-17.7558, 140.9959) (-16.603, 140.9959) knots 0 0 0 1 1 1
  spline S117 degree 2 poles (-16.603, 140.9959) (-15.4025, 140.9959) (-14.8533, 141.4359) knots 0 0 0 1 1 1
  spline S118 degree 2 poles (-14.8533, 141.4359) (-14.3042, 141.8759) (-14.3042, 142.4966) knots 0 0 0 1 1 1
  spline S119 degree 2 poles (-14.3042, 142.4966) (-14.3042, 143.0355) (-14.693, 143.3834) knots 0 0 0 1 1 1
  spline S120 degree 2 poles (-14.693, 143.3834) (-15.075, 143.7312) (-16.6883, 144.0962) knots 0 0 0 1 1 1
  spline S121 degree 2 poles (-16.6883, 144.0962) (-18.3015, 144.4611) (-18.9018, 144.734) knots 0 0 0 1 1 1
  spline S122 degree 2 poles (-18.9018, 144.734) (-19.7749, 145.1364) (-20.191, 145.7538) knots 0 0 0 1 1 1
  spline S123 degree 2 poles (-20.191, 145.7538) (-20.6071, 146.3711) (-20.6071, 147.176) knots 0 0 0 1 1 1
  spline S124 degree 2 poles (-20.6071, 147.176) (-20.6071, 147.9741) (-20.1501, 148.6801) knots 0 0 0 1 1 1
  spline S125 degree 2 poles (-20.1501, 148.6801) (-19.693, 149.3861) (-18.837, 149.7783) knots 0 0 0 1 1 1
  spline S126 degree 2 poles (-18.837, 149.7783) (-17.9809, 150.1705) (-16.91, 150.1705) knots 0 0 0 1 1 1
  spline S127 degree 2 poles (-16.91, 150.1705) (-15.5525, 150.1705) (-14.6351, 149.7749) knots 0 0 0 1 1 1
  spline S128 degree 2 poles (-14.6351, 149.7749) (-13.7176, 149.3793) (-13.1958, 148.5846) knots 0 0 0 1 1 1
  spline S129 degree 2 poles (-13.1958, 148.5846) (-12.6739, 147.7899) (-12.6467, 146.7872) knots 0 0 0 1 1 1
extrude "Extrude7" cut sketch "Sketch7" against normal blind 3 contours L50 L51 S55 S56 S57 S58 S59 S60 S61 S62 S63 S64 S65 L52 | L59 L60 L61 L62 L63 L64 L65 L66 L67 L68 L69 L70 | L71 L72 L73 L74 L75 L76 L77 L78 | L82 L83 S81 S82 S83 S84 S85 S86 S87 L84 L85 L86 S88 S89 S90 S91 L87 L88 L89 | L93 S97 S98 S99 S100 S101 S102 S103 S104 S105 S106 S107 S108 S109 S110 S111 S112 S113 S114 L94 S115 S116 S117 S118 S119 S120 S121 S122 S123 S124 S125 S126 S127 S128 S129 bodies 6 makes body 11 at (-22.0759, 0, 147.6739) makes body 12 at (-22.2897, 0, 143.1946) makes body 13 at (6.3552, 0, 142.2078) makes body 14 at (46.8309, 0, 145.9837)
